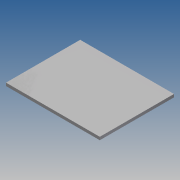
# Autodesk Inventor part: Ground
Saved by Autodesk Inventor 2016 (Build 200138000, 138)
## iProperties
Created: 2014-06-12
Part Number: Ground
Material: Acier
Document SubType Name: Modeling
Designer: Yann
Mass: 50526 g
Surface Area: 6893.39 cm^2
Volume: 6436.43 cm^3
Density: 7.85 g/cm^3
Appearance: Acier
Author: Yann
Autodesk Inventor part; units mm, degrees
ref_plane "YZ Plane" through (0, 0, 0) normal (1, 0, 0) x (0, 1, 0)
ref_plane "XZ Plane" through (0, 0, 0) normal (0, 1, 0) x (-1, 0, 0)
ref_plane "XY Plane" through (0, 0, 0) normal (0, 0, 1) x (1, 0, 0)
sketch "Esquisse1" plane through (0, 0, 0) normal (0, 0, 1) x (1, 0, 0)
  line L0 (-318.9478, -252.2526) -> (318.9478, -252.2526)
  line L1 (318.9478, -252.2526) -> (318.9478, 252.2526)
  line L2 (318.9478, 252.2526) -> (-318.9478, 252.2526)
  line L3 (-318.9478, 252.2526) -> (-318.9478, -252.2526)
  line L4 (-318.9478, -252.2526) -> (318.9478, 252.2526) construction
  line L5 (318.9478, -252.2526) -> (-318.9478, 252.2526) construction
  point P0 (0, 0)
  constraints: 12 end point, 2 midpoint, 2 parallel, 1 horizontal, 1 perpendicular
extrude "Extrusion1" add sketch "Esquisse1" along normal blind 20
